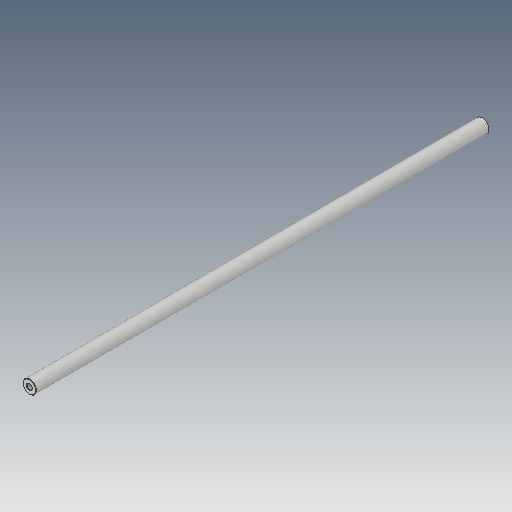
# Autodesk Inventor part: BaseSlide_p10ALshaft
Saved by Autodesk Inventor 2019.4 (Build 234330000, 330)
## iProperties
Created: 2019-07-02
Part Number: BaseSlide_p10ALshaft
Material: アルミニウム 2014-T6
Document SubType Name: Modeling
Designer: AzLIer
Density: 2.78927 g/cm^3
Appearance: サテン
Author: AzLIer
Autodesk Inventor part; units mm, degrees
ref_plane "YZ Plane" through (0, 0, 0) normal (1, 0, 0) x (0, 1, 0)
ref_plane "XZ Plane" through (0, 0, 0) normal (0, 1, 0) x (-1, 0, 0)
ref_plane "XY Plane" through (0, 0, 0) normal (0, 0, 1) x (1, 0, 0)
sketch "スケッチ1" plane through (0, 0, 0) normal (0, 0, 1) x (1, 0, 0)
  circle A0 centre (0, 0) radius 5
  dimension "d0" = 10
  constraints: 1 centre point, 1 coincident
  measures "d0" diameter of A0
extrude "押し出し1" add sketch "スケッチ1" along normal blind 340
sketch "スケッチ2" plane through (0, 0, 340) normal (0, 0, 1) x (1, 0, 0)
  point P0 (0, 0)
sketch "スケッチ3" plane through (0, 0, 0) normal (0, 0, -1) x (-1, 0, 0)
  point P0 (0, 0)
hole "穴1" at (0, 0, 340) direction (0, 0, -1) diameter 4.134 depth 30 tip angle 118 thread size "M5x0.8" class "6H" standard "ISO Metric profile"
hole "穴2" at (0, 0, 0) direction (0, 0, 1) diameter 4.134 depth 30 tip angle 118 thread size "M5x0.8" class "6H" standard "ISO Metric profile"
chamfer "面取り1" distance 0.3 angle 45 4 edges at (-5, 0, 340) (-5, 0, 0) (0, 2.067, 340) (0, -2.067, 0)
